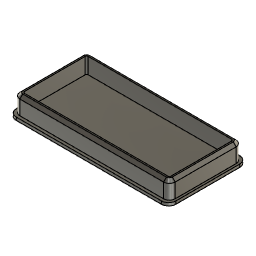
DuctEndCap (Autodesk Fusion 360 design; units mm, degrees)
Autodesk Fusion 360 part; units mm, degrees
sketch "Sketch1" plane through (0, 0, 0) normal (0, 0, 1) x (1, 0, 0) in component "Component"
  line L0 (53.5, -25) -> (-53.5, -25)
  line L1 (-53.5, -25) -> (-53.5, 25)
  line L2 (-53.5, 25) -> (53.5, 25)
  line L3 (53.5, 25) -> (53.5, -25)
  line L4 (53.5, -25) -> (-53.5, 25) construction
  line L5 (-53.5, -25) -> (53.5, 25) construction
  dimension "d1" = 50
  dimension "d2" = 107
  constraint perpendicular L0 L1
  constraint parallel L0 L2
  constraint parallel L1 L3
  constraint horizontal L0
  constraint coincident L4 origin
  constraint coincident L5 origin
  measures "d1" distance of L0.end L1.end
  measures "d2" distance of L1.end L2.end
extrude "Extrude1" add sketch "Sketch1" along normal blind 12 in component "Component"
sketch "Sketch2" plane through (0, 0, 0) normal (0, 0, -1) x (1, 0, 0) in component "Component"
  line L0 (-53.5, -25) -> (53.5, -25)
  line L1 (53.5, -25) -> (53.5, 25)
  line L2 (53.5, 25) -> (-53.5, 25)
  line L3 (-53.5, 25) -> (-53.5, -25)
  line L4 (55, -27) -> (-55, -27)
  line L5 (-55, -27) -> (-55, 27)
  line L6 (-55, 27) -> (55, 27)
  line L7 (55, 27) -> (55, -27)
  line L8 (55, -27) -> (-55, 27) construction
  line L9 (-55, -27) -> (55, 27) construction
  dimension "d5" = 54
  dimension "d6" = 110
  constraint perpendicular L4 L5
  constraint parallel L4 L6
  constraint parallel L5 L7
  constraint horizontal L4
  constraint coincident L8 origin
  constraint coincident L9 origin
  measures "d5" distance of L4.end L5.end
  measures "d6" distance of L5.end L6.end
extrude "Extrude2" add sketch "Sketch2" along normal blind 2 contours L0 L1 L2 L3 | L4 L5 L6 L7 in component "Component"
fillet "Fillet1" radius 5 4 edges at (-55, -27, -1) (-55, 27, -1) (55, 27, -1) (55, -27, -1) in component "Component"
fillet "Fillet2" radius 4 4 edges at (53.5, 25, 6) (53.5, -25, 6) (-53.5, -25, 6) (-53.5, 25, 6) in component "Component"
shell "Shell1" thickness 3 removed faces 1 at (-16.5, -8.3333, 12) in component "Component"
chamfer "Chamfer1" distance 2 angle 45 8 edges at (52.3284, -23.8284, 12) (53.5, 0, 12) (52.3284, 23.8284, 12) (0, 25, 12) (-52.3284, 23.8284, 12) (-53.5, 0, 12) (-52.3284, -23.8284, 12) (0, -25, 12) in component "Component"
component "Component" placed x (1, 0, 0) y (0, 1, 0) z (0, 0, 1) at (0, 0, 0)
